lego-tray-corner-right (Autodesk Fusion 360 design; units mm, degrees)
Autodesk Fusion 360 part; units mm, degrees
note: some values were not read from the file. Set by a fixed rule: which sketch regions a step uses.
sketch "Sketch1" plane through (0, 0, 0) normal (0, 1, 0) x (1, 0, 0)
  line L0 (0, 0) -> (-82.2706, 0)
  line L1 (-82.2706, 0) -> (-82.2706, 65.5066)
  line L2 (-20.3962, 127.381) -> (0, 127.381)
  line L3 (0, 127.381) -> (0, 0)
  arc A0 (-20.3962, 127.381) -> (-82.2706, 65.5066) centre (-20.3962, 65.5066) ccw
  line L4 (-81.8896, 0.381) -> (-81.8896, 65.5066)
  arc A1 (-20.3962, 127) -> (-81.8896, 65.5066) centre (-20.3962, 65.5066) ccw
  line L5 (-20.3962, 127) -> (-0.381, 127)
  line L6 (-0.381, 127) -> (-0.381, 0.381)
  line L7 (-0.381, 0.381) -> (-81.8896, 0.381)
  dimension "d1" = 82.2706
  dimension "d2" = 127.381
  dimension "d3" = 61.8744
  dimension "d27" = -0.381
  constraint horizontal L0
  constraint vertical L1
  constraint horizontal L2
  constraint vertical L3
  constraint coincident L0.start L3.end
  constraint tangent L1 A0
  constraint tangent L2 A0
  measures "d1" distance of L0.start L0.end
  measures "d2" distance of L0.start L2.end
  measures "d3" radius of A0
extrude "Extrude1" add sketch "Sketch1" along normal blind 76.2 contours L4 A1 L5 L6 L7 makes body 1
draft "Draft1" angle -4 neutral plane through (0, 0, 0) pull (0, 1, 0) 3 faces at (-81.8896, 25.4, -22.0895) (-81.8199, 50.8, -68.4326) (-13.7245, 25.4, -127) on bodies 1
fillet "Fillet1" radius 6.35 3 edges at (-0.381, 38.1, -129.6642) (-0.381, 38.1, -0.381) (-84.5538, 38.1, -0.381) on bodies 1
fillet "Fillet2" radius 3.175 8 edges at (-0.381, 0, -63.6827) (-2.2409, 0, -125.1356) (-13.5636, 0, -127) (-63.8786, 0, -108.989) (-81.8896, 0, -36.1188) (-80.0252, 0, -2.2409) (-41.1275, 0, -0.381) (-2.2409, 0, -2.2409) on bodies 1
shell "Shell1" thickness 1.524 removed faces 1 at (-28.4244, 76.2, -72.3421) on bodies 1
mirror "Mirror1" about plane through (0, 0, 0) normal (1, 0, 0) of bodies 1 makes body 2
delete_body "RemoveBody1" bodies 1
sketch "Sketch2" plane through (0, 76.2, 0) normal (0, 1, 0) x (-1, 0, 0)
  line L0 (-19.431, -1.905) -> (-38.481, -1.905)
  line L1 (-38.481, -1.905) -> (-38.481, -0.381)
  line L2 (-38.481, -0.381) -> (-19.431, -0.381)
  line L3 (-19.431, -0.381) -> (-19.431, -1.905)
  line L4 (-0.381, -68.8129) -> (-1.905, -68.8129)
  line L5 (-1.905, -68.8129) -> (-1.905, -113.2629)
  line L6 (-1.905, -113.2629) -> (-0.381, -113.2629)
  line L7 (-0.381, -113.2629) -> (-0.381, -68.8129)
  line L8 (-0.381, -6.731) -> (-0.381, -125.9629)
  line L9 (-1.905, -125.9629) -> (-1.905, -6.731)
  line L10 (-6.731, -1.905) -> (-80.8525, -1.905)
  line L11 (-80.8525, -0.381) -> (-6.731, -0.381)
  dimension "d17" = 19.05
  dimension "d18" = 44.45
  dimension "d32" = 12.7
  dimension "d33" = 12.7
  constraint horizontal L0
  constraint vertical L1
  constraint horizontal L2
  constraint vertical L3
  constraint horizontal L4
  constraint vertical L5
  constraint horizontal L6
  constraint vertical L7
  constraint coincident L0.end L10
  constraint coincident L2.end L11
  constraint coincident L5.end L9
  constraint coincident L4.start L8
  measures "d17" distance of L1.end L2.end
  measures "d18" distance of L4.start L6.end
  measures "d32" distance of L2.end L11.end
  measures "d33" distance of L6.end L8.end
extrude "Extrude2" cut sketch "Sketch2" against normal blind 12.7 bodies 2
draft "Draft2" angle 30 neutral plane through (0, 63.5, 0) pull (0, 1, 0) 4 faces at (38.481, 67.7333, -1.397) (1.397, 67.7333, -113.2629) (0.889, 67.7333, -68.8129) (19.431, 67.7333, -0.889) on bodies 2
fillet "Fillet3" radius 6.35 8 edges at (1.143, 76.2, -120.5953) (1.143, 63.5, -113.2629) (1.143, 76.2, -61.4806) (1.143, 63.5, -68.8129) (12.0987, 76.2, -1.143) (19.431, 63.5, -1.143) (38.481, 63.5, -1.143) (45.8133, 76.2, -1.143) on bodies 2
